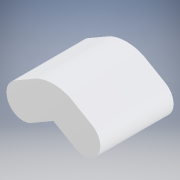
# Autodesk Inventor part: SA001
Saved by Autodesk Inventor 2017 SP1 (Build 210196100, 196)
## iProperties
Created: 2017-06-05
Part Number: SA001
Material: ABS Plastic
Document SubType Name: Modeling
Designer: Zach
Density: 1.06 g/cm^3
Appearance: CR White
Author: Zach
Autodesk Inventor part; units mm, degrees
ref_plane "YZ Plane" through (0, 0, 0) normal (1, 0, 0) x (0, 1, 0)
ref_plane "XZ Plane" through (0, 0, 0) normal (0, 1, 0) x (-1, 0, 0)
ref_plane "XY Plane" through (0, 0, 0) normal (0, 0, 1) x (1, 0, 0)
sketch "Sketch3" plane through (0, 0, 0) normal (0, 0, 1) x (1, 0, 0)
  circle A0 centre (0, -206.2159) radius 225 construction
  line L0 (-90, 0) -> (90, 0) construction
  circle A1 centre (-166.2436, -147.9423) radius 90 construction
  circle A2 centre (166.2436, -147.9423) radius 90 construction
  line L1 (-90, 0) -> (-211.2436, -70) construction
  line L2 (-90, 0) -> (0, -155.8846) construction
  line L3 (0, -155.8846) -> (90, 0) construction
  line L4 (0, -155.8846) -> (-121.2436, -225.8846) construction
  line L5 (90, 0) -> (211.2436, -70) construction
  line L6 (0, -155.8846) -> (121.2436, -225.8846) construction
  arc A3 (-211.2436, -70) -> (-121.2436, -225.8846) centre (-166.2436, -147.9423) ccw
  arc A4 (121.2436, -225.8846) -> (211.2436, -70) centre (166.2436, -147.9423) ccw
  line L7 (-211.2436, -70) -> (-90, 0)
  line L8 (-121.2436, -225.8846) -> (0, -155.8846)
  line L9 (121.2436, -225.8846) -> (0, -155.8846)
  line L10 (90, 0) -> (211.2436, -70)
  arc A5 (90, 0) -> (-90, 0) centre (0, -206.2159) ccw
  point P0 (0, 0)
  point P1 (0, 0)
  dimension "d10" = 450
  dimension "d11" = 180
  dimension "d12" = 180
  dimension "d13" = 180
  dimension "d15" = 140
  dimension "d16" = 180
  dimension "d17" = 140
  dimension "d18" = 90
  dimension "d19" = 90
  dimension "d20" = 140
  dimension "d21" = 140
  dimension "d23" = 90
  constraints: 22 end point, 13 point on circle, 6 centre point, 3 tangent, 2 coincident, 2 collinear, 2 vertical alignment, 1 concentric, 1 horizontal, 1 horizontal alignment, 1 midpoint
  measures "d10" diameter of A0
  measures "d11" distance of L0.start L0.end
  measures "d12" diameter of A1
  measures "d13" diameter of A2
  measures "d15" distance of L0.start L1.end
  measures "d16" distance of L0.start L2.end
  measures "d17" distance of L2.end L4.end
  measures "d18" angle of L2 L1
  measures "d19" angle of L2 L4
  measures "d20" distance of L0.end L5.end
  measures "d21" distance of L2.end L6.end
  measures "d23" angle of L5 L3
extrude "Extrusion3" add sketch "Sketch3" along normal blind 400
body "Solid2"
